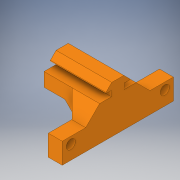
# Autodesk Inventor part: 20X20 lift conecter
Saved by Autodesk Inventor 2019 (Build 230136000, 136)
## iProperties
Created: 2018-10-23
Part Number: 20X20 lift conecter
Material: PC/ABS Plastic
Document SubType Name: Modeling
Designer: User
Density: 0.357273 g/cm^3
Appearance: Orange
Mass: 2.99758 g
Surface Area: 36.2331 cm^2
Volume: 8.39019 cm^3
Author: User
Autodesk Inventor part; units mm, degrees
ref_plane "YZ Plane" through (0, 0, 0) normal (1, 0, 0) x (0, 1, 0)
ref_plane "XZ Plane" through (0, 0, 0) normal (0, 1, 0) x (-1, 0, 0)
ref_plane "XY Plane" through (0, 0, 0) normal (0, 0, 1) x (1, 0, 0)
sketch "Sketch1" plane through (0, 0, 0) normal (0, 1, 0) x (-1, 0, 0)
  line L0 (2.54, 0.2286) -> (4.953, 0.2286)
  line L1 (4.953, 0.2286) -> (4.953, -16.4084)
  line L2 (4.953, -16.4084) -> (2.54, -16.4084)
  line L3 (2.54, -5.1689) -> (7.493, -5.1689)
  line L4 (7.493, -5.1689) -> (7.493, -11.0109)
  line L5 (7.493, -11.0109) -> (2.54, -11.0109)
  line L6 (10.5664, -5.3213) -> (10.5664, -10.8585)
  line L7 (7.493, -13.9319) -> (7.493, -2.2479)
  line L8 (7.493, -13.9319) -> (10.5664, -10.8585)
  line L9 (7.493, -2.2479) -> (10.5664, -5.3213)
  line L10 (2.54, -16.4084) -> (2.54, 0.2286)
  point P0 (0, 0)
  dimension "d1" = 16.637
  dimension "d2" = 2.54
  dimension "d9" = 3.0734
  dimension "d12" = 0
  dimension "d16" = 11.684
  dimension "d20" = 135
  dimension "d21" = 135
  dimension "d26" = 2.921
  dimension "d38" = 5.5372
  dimension "d77" = 5.842
  dimension "d78" = 5.3975
  constraints: 22 end point, 3 parallel, 2 horizontal, 2 perpendicular, 2 point on line
  measures "d1" distance of L0.end L1.end
  measures "d2" distance between parallel lines of L4 L1
  measures "d9" distance between parallel lines of L6 L7
  measures "d12" distance between parallel lines of L4 L7
  measures "d16" distance of L7.start L7.end
  measures "d20" angle of L8 L6
  measures "d21" angle of L9 L6
  measures "d26" distance from line of L3 L7.end
  measures "d38" distance of L6.start L6.end
  measures "d77" distance between parallel lines of L5 L3
  measures "d78" distance between parallel lines of L2 L5
extrude "Extrusion2" add sketch "Sketch1" along normal blind 25.4
fillet "Fillet1" radius 0.254 2 edges at (-7.493, 12.7, -13.9319) (-7.493, 12.7, -2.2479)
thicken "Thicken1" operation add thickness 3.81 both sides no extend neighbours yes toward (1, 0, 0) faces at (-2.54, 8.4667, -5.3171)
sketch "Sketch2" plane through (0, 25.4, 0) normal (0, 1, 0) x (1, 0, 0)
  line L0 (-4.953, 5.1689) -> (-4.953, -0.2286) projected
  line L1 (-4.953, 16.4084) -> (-4.953, 11.0109) projected
  line L2 (-4.953, -0.2286) -> (10.922, -0.2286)
  line L3 (10.922, -0.2286) -> (10.922, 16.4084)
  line L4 (10.922, 16.4084) -> (-4.953, 16.4084)
  line L5 (-4.953, 16.4084) -> (-4.953, -0.2286)
  point P0 (0, 0)
  dimension "d46" = 15.875
  constraints: 8 end point, 2 parallel, 1 horizontal, 1 perpendicular
  measures "d46" distance of L4.end L3.end
extrude "Extrusion3" add sketch "Sketch2" against normal blind 6.35
sketch "Sketch3" plane through (0, 25.4, 0) normal (0, 1, 0) x (1, 0, 0)
  line L0 (1.397, -17.3101) -> (10.922, -17.3101)
  line L1 (10.922, -17.3101) -> (10.922, 33.4899)
  line L2 (10.922, 33.4899) -> (1.397, 33.4899)
  line L3 (1.397, 33.4899) -> (1.397, -17.3101)
  line L4 (10.922, -0.2286) -> (10.922, 16.4084) projected
  line L5 (-4.953, 11.0109) -> (-7.493, 11.0109) projected
  line L6 (-7.493, 11.0109) -> (-7.493, 13.3187) projected
  arc A0 (-7.493, 13.3187) -> (-7.9266, 13.4983) centre (-7.747, 13.3187) ccw projected
  line L7 (-7.9266, 13.4983) -> (-10.5664, 10.8585) projected
  line L8 (-10.5664, 10.8585) -> (-10.5664, 5.3213) projected
  line L9 (-10.5664, 5.3213) -> (-7.9266, 2.6815) projected
  arc A1 (-7.9266, 2.6815) -> (-7.493, 2.8611) centre (-7.747, 2.8611) ccw projected
  line L10 (-7.493, 2.8611) -> (-7.493, 5.1689) projected
  line L11 (-7.493, 5.1689) -> (-4.953, 5.1689) projected
  line L12 (-4.953, 5.1689) -> (-4.953, -0.2286) projected
  line L13 (-4.953, -0.2286) -> (10.922, -0.2286) projected
  line L14 (10.922, -0.2286) -> (10.922, 16.4084) projected
  line L15 (10.922, 16.4084) -> (-4.953, 16.4084) projected
  line L16 (-4.953, 16.4084) -> (-4.953, 11.0109) projected
  point P0 (0, 0)
  dimension "d49" = 50.8
  dimension "d50" = 16.637
  dimension "d51" = 17.0815
  dimension "d52" = 9.525
  constraints: 8 end point, 2 parallel, 1 collinear, 1 horizontal, 1 perpendicular
  measures "d49" distance of L0.end L1.end
  measures "d50" distance between parallel lines of L15 L13
  measures "d51" distance between parallel lines of L13 L0
  measures "d52" distance of L1.end L2.end
extrude "Extrusion4" add sketch "Sketch3" against normal blind 6.35 contours L3 L13 L1 L0 | L3 L15 L1 L13 | L3 L2 L1 L15
chamfer "Chamfer1" distance 6.35 angle 45 2 edges at (1.397, 22.225, 0.2286) (1.397, 22.225, -16.4084)
sketch "Sketch4" plane through (0, 25.4, 0) normal (0, 1, 0) x (1, 0, 0)
  line L0 (1.397, -17.3101) -> (10.922, -17.3101) projected
  line L1 (10.922, -17.3101) -> (10.922, 33.4899) projected
  line L2 (10.922, 33.4899) -> (1.397, 33.4899) projected
  line L3 (0.635, 26.162) -> (0.635, 33.4899) projected
  line L4 (0.635, -17.3101) -> (0.635, -9.525) projected
  point P0 (0, 0)
  point P1 (4.5466, -13.3985)
  point P2 (4.5466, 29.5783)
  point P3 (0.635, -9.525)
  dimension "d64" = 3.9116
  dimension "d66" = 3.9116
  dimension "d75" = 3.9116
  dimension "d76" = 3.9116
  measures "d64" distance from line of L0 point (4.547, -13.398)
  measures "d66" distance from line of L2 point (4.547, 29.578)
  measures "d75" distance from line of L3 point (4.547, 29.578)
  measures "d76" distance from line of L4 point (4.547, -13.398)
hole "Hole1" at (4.5466, 25.4, 13.3985) at (4.5466, 25.4, -29.5783) direction (0, -1, 0) diameter 4.191 end through all
sketch "Sketch5" plane through (0, 0, 0) normal (0, -1, 0) x (1, 0, 0)
  line L0 (-4.953, -16.4084) -> (1.27, -22.6314) projected
  line L1 (-4.953, -16.4084) -> (2.7797, -16.4084)
  line L2 (2.7797, -16.4084) -> (2.7797, -25.516)
  line L3 (2.7797, -25.516) -> (-4.953, -25.516)
  line L4 (-4.953, -25.516) -> (-4.953, -16.4084)
  line L5 (-4.953, -5.1689) -> (-4.953, 0.2286) projected
  line L6 (-4.953, 0.2286) -> (4.8466, 0.2286)
  line L7 (4.8466, 0.2286) -> (4.8466, 7.7688)
  line L8 (4.8466, 7.7688) -> (-4.953, 7.7688)
  line L9 (-4.953, 7.7688) -> (-4.953, 0.2286)
  point P0 (0, 0)
  constraints: 16 end point, 4 parallel, 2 horizontal, 2 perpendicular
extrude "Extrusion5" cut sketch "Sketch5" against normal blind 19.05
chamfer "Chamfer4" distance 6.1976 angle 45 2 edges at (-1.8415, 19.05, 0.2286) (-1.8415, 19.05, -16.4084)
chamfer "Chamfer5" distance 9.525 angle 45 3 edges at (1.27, 19.05, 3.3274) (1.27, 19.05, -8.0899) (1.27, 19.05, -19.5072)
equation "\"d21\" = d20"
body "Solid2"
